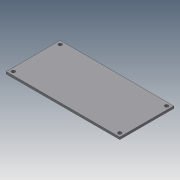
# Autodesk Inventor part: Part4
Saved by Autodesk Inventor 2014 SP1 (Build 180222100, 222)
## iProperties
Created: 2015-04-02
Part Number: Part4
Material: Generic
Document SubType Name: Modeling
Designer: tom
Density: 1 g/cm^3
Appearance: Default
Author: tom
Autodesk Inventor part; units mm, degrees
ref_plane "YZ Plane" through (0, 0, 0) normal (1, 0, 0) x (0, 1, 0)
ref_plane "XZ Plane" through (0, 0, 0) normal (0, 1, 0) x (-1, 0, 0)
ref_plane "XY Plane" through (0, 0, 0) normal (0, 0, 1) x (1, 0, 0)
sketch "Sketch1" plane through (0, 0, 0) normal (0, 1, 0) x (-1, 0, 0)
  line L0 (40, -19) -> (-40, -19)
  line L1 (-40, -19) -> (-40, 19)
  line L2 (-40, 19) -> (40, 19)
  line L3 (40, 19) -> (40, -19)
  line L4 (37.5, -16.5) -> (-37.5, -16.5) construction
  line L5 (-37.5, -16.5) -> (-37.5, 16.5) construction
  line L6 (-37.5, 16.5) -> (37.5, 16.5) construction
  line L7 (37.5, 16.5) -> (37.5, -16.5) construction
  circle A0 centre (37.5, -16.5) radius 1.25
  line L8 (0, -19) -> (0, 19) construction
  line L9 (-40, 0) -> (40, 0) construction
  circle A1 centre (-37.5, -16.5) radius 1.25
  circle A2 centre (37.5, 16.5) radius 1.25
  circle A3 centre (-37.5, 16.5) radius 1.25
  point P0 (0, 0)
  dimension "d0" = 80
  dimension "d1" = 38
  dimension "d2" = 40
  dimension "d3" = 19
  dimension "d4" = 75
  dimension "d5" = 33
  dimension "d6" = 2.5
  dimension "d7" = 2.5
  dimension "d8" = 2.5
  constraints: 20 end point, 4 centre point, 4 midpoint, 4 parallel, 3 symmetric about line, 2 horizontal, 2 perpendicular, 1 coincident, 3 other
  measures "d0" distance of L1.end L2.end
  measures "d1" distance of L0.end L1.end
  measures "d2" distance from line of L3 point (0, 0)
  measures "d3" distance from line of L2 point (0, 0)
  measures "d4" distance of L5.end L6.end
  measures "d5" distance of L4.end L5.end
  measures "d6" distance between parallel lines of L0 L4
  measures "d7" distance between parallel lines of L3 L7
  measures "d8" diameter of A0
extrude "Extrusion1" add sketch "Sketch1" along normal blind 1.5875
equation "\"d2\" = 0.5 * d0"
equation "\"d3\" = 0.5 * d1"
equation "\"d7\" = d6"
body "Solid1"
